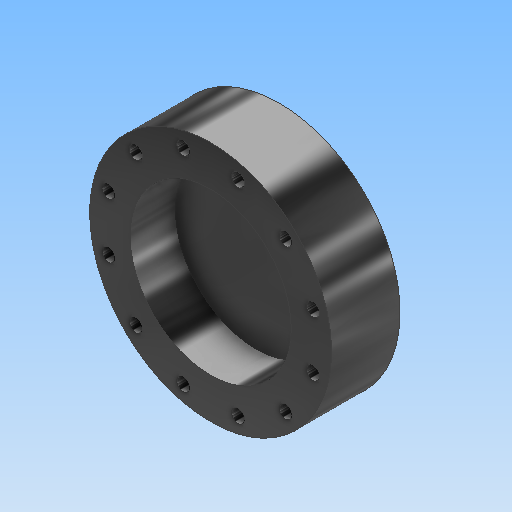
# Autodesk Inventor part: XL200 PART1
Saved by Autodesk Inventor 2020.1 (Build 241239000, 239)
## iProperties
Created: 2001-03-07
Part Number: XL200 PART1
Document SubType Name: Modeling
Designer: Joe M
Material: Steel, Mild
Engineer: Joe M
Density: 7.86 g/cm^3
Appearance: Chrome - Polished Black
Control State: 0
Master: False
Checked Out: False
Shininess: 20.0
Length Units: 11269
Angle Units: 11279
Time Units: 11290
Mass Units: 11283
Length Display Precision: 3
Angle Display Precision: 2
Compacted: True
Density: 0.0
Volumn: 0.0
Area: 0.0
PropertySet Name: Model Information
Author: Joe M
Autodesk Inventor part; units mm, degrees
ref_plane "YZ Plane" through (0, 0, 0) normal (1, 0, 0) x (0, 1, 0)
ref_plane "XZ Plane" through (0, 0, 0) normal (0, 1, 0) x (-1, 0, 0)
ref_plane "XY Plane" through (0, 0, 0) normal (0, 0, 1) x (1, 0, 0)
sketch "Sketch1" plane through (-446.9925, -258.9913, -45) normal (0, 0, 1) x (1, 0, 0)
  point P0 (521.2387, 184.7451)
sketch "Sketch2" plane through (-446.9925, -258.9913, -45) normal (0, 0, 1) x (1, 0, 0)
  circle A0 centre (446.9925, 258.9913) radius 120
  dimension "d43" = 240
  constraints: 1 centre point, 1 other
  measures "d43" diameter of A0
extrude "ExtrusionBlind1" add sketch "Sketch2" along normal blind 90
sketch "Sketch3" plane through (-446.9925, -258.9913, -45) normal (0, 0, 1) x (1, 0, 0)
  circle A0 centre (446.9925, 258.9913) radius 143.9167
  circle A1 centre (446.9925, 258.9913) radius 90
  circle A2 centre (446.9925, 258.9913) radius 120 projected
  dimension "d44" = 287.8334
  dimension "d45" = 180
  constraints: 2 centre point, 1 coincident, 1 concentric
  measures "d44" diameter of A0
  measures "d45" diameter of A1
extrude "ExtrusionBlind2" cut sketch "Sketch3" along normal blind 22 contours A0 | A2
hole "Hole1" at (74.2462, -74.2462, -45) direction (0, 0, 1) diameter 13 end through all
pattern_circular "PolarArray1" count 12 over 360 about axis through (0, 0, -45) along (0, 0, 1) of "Hole1", "Hole1"
sketch "Sketch6" plane through (0, 0, -45) normal (0, 0, -1) x (-1, 0, 0)
  point P0 (0, -30)
sketch "Sketch7" plane through (0, 0, -45) normal (0, 0, -1) x (-1, 0, 0)
  point P0 (-22.5, 5.5)
sketch "Sketch8" plane through (0, 0, 45) normal (0, 0, 1) x (1, 0, 0)
  circle A0 centre (0, 0) radius 80
  circle A1 centre (0, 0) radius 120 projected
  dimension "d42" = 160
  constraints: 3 other
  measures "d42" diameter of A0
extrude "ExtrusionBlind3" cut sketch "Sketch8" against normal blind 45 contours A0
chamfer "Chamfer1" distance 10 angle 45 1 edges at (-90, 0, -45)
hole "Hole2" at (0, -30, -45) direction (0, 0, 1) diameter 10 depth 20 tip angle 118
hole "Hole3" [suppressed]
sketch "Sketch12" plane through (0, 0, -45) normal (0, 0, -1) x (-1, 0, 0)
  line L0 (-2, -119.5) -> (-2, -141.4896)
  line L1 (-2, -141.4896) -> (2, -141.4896)
  line L2 (2, -119.5) -> (2, -141.4896)
  line L3 (2, -119.5) -> (-2, -119.5)
  dimension "d46" = 4
  dimension "d47" = 21.9896
  constraints: 8 end point, 2 horizontal, 2 vertical
  measures "d46" distance between parallel lines of L2 L0
  measures "d47" distance between parallel lines of L3 L1
extrude "ExtrusionThru1" cut sketch "Sketch12" against normal through all
body "Solid1"
